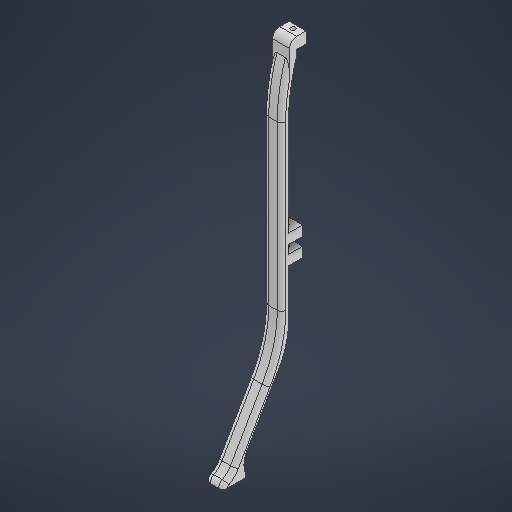
# Autodesk Inventor part: podpory
Saved by Autodesk Inventor 2026.2 (Build 302298010, 298A)
## iProperties
Created: 2026-04-19
Part Number: podpory
Material: Ogólny
Document SubType Name: Modeling
Designer: macie
Density: 1 g/cm^3
Appearance: Domyślna
Author: macie
Autodesk Inventor part; units mm, degrees
ref_plane "YZ Plane" through (0, 0, 0) normal (1, 0, 0) x (0, 1, 0)
ref_plane "XZ Plane" through (0, 0, 0) normal (0, 1, 0) x (-1, 0, 0)
ref_plane "XY Plane" through (0, 0, 0) normal (0, 0, 1) x (1, 0, 0)
sketch "Szkic1" plane through (0, 0, 0) normal (1, 0, 0) x (0, 1, 0)
  line L0 (0, 100.074) -> (0, 95.074)
  line L1 (0, 95.074) -> (5, 95.074)
  line L2 (5, 95.074) -> (5, 100.074)
  line L3 (5, 100.074) -> (0, 100.074)
  line L4 (178.8725, 94.2545) -> (173.8725, 94.2545)
  line L5 (173.8725, 94.2545) -> (173.8725, 89.2545)
  line L6 (173.8725, 89.2545) -> (178.8725, 89.2545)
  line L7 (178.8725, 89.2545) -> (178.8725, 94.2545)
  line L8 (5, 95.074) -> (137.3058, 95.074)
  arc A0 (173.8725, 89.2545) -> (137.3058, 95.074) centre (135.3654, -34.9115) ccw
  line L9 (5, 100.074) -> (137.3058, 100.074)
  arc A1 (173.8725, 94.2545) -> (137.3058, 100.074) centre (136.1596, -24.9207) ccw
  point P0 (0, 0)
  dimension "d0" = 95.074
  dimension "d1" = 5
  dimension "d2" = 5
  dimension "d4" = 0
  dimension "d5" = 89.2545
  dimension "d6" = 130
  dimension "d8" = 5
  dimension "d9" = 5
  dimension "d10" = 125
  dimension "d11" = 24.9207
  dimension "d12" = 34.9115
  dimension "d13" = 136.1596
  constraints: 20 end point, 4 parallel, 4 point on circle, 3 horizontal, 2 centre point, 2 perpendicular, 1 vertical
  measures "d0" distance from line of point (0, 0) L1
  measures "d1" distance between parallel lines of L1 L3
  measures "d2" distance between parallel lines of L0 L2
  measures "d4" distance from line of point (0, 0) L0
  measures "d5" distance from line of point (0, 0) L6
  measures "d6" radius of A0
  measures "d8" distance between parallel lines of L5 L7
  measures "d9" distance between parallel lines of L6 L4
  measures "d10" radius of A1
  measures "d11" vertical distance of point (0, 0) A1.centre
  measures "d12" vertical distance of point (0, 0) A0.centre
  measures "d13" horizontal distance of point (0, 0) A1.centre
extrude "Wyciągnięcie proste1" add sketch "Szkic1" along normal blind 12
sketch "Szkic2" plane through (0, 173.8725, 89.2545) normal (0, 0, -1) x (-1, 0, 0)
  line L0 (0, 0) -> (-12, 0) projected
  line L1 (0, 0) -> (-12, 0)
  line L2 (-12, 0) -> (-12, 12)
  line L3 (-12, 12) -> (0, 12)
  line L4 (0, 12) -> (0, 0)
  line L5 (-12, 0) -> (0, 0)
  line L6 (0, 0) -> (0, 4)
  line L7 (0, 4) -> (-12, 4)
  line L8 (-12, 4) -> (-12, 0)
  point P0 (0, -173.8725)
  point P1 (-12, 4)
  dimension "d16" = 12
  dimension "d17" = 12
  dimension "d18" = 4
  constraints: 16 end point, 4 parallel, 2 horizontal, 2 perpendicular, 1 point on line
  measures "d16" distance between parallel lines of L4 L2
  measures "d17" distance between parallel lines of L0 L3
  measures "d18" distance between parallel lines of L0 L7
extrude "Wyciągnięcie proste2" add sketch "Szkic2" along normal blind 6.653 and the other way blind 5 contours L7 L2 L3 L4
sketch "Szkic3" plane through (0, 177.8725, 89.2545) normal (0, -1, 0) x (1, 0, 0)
  line L0 (12, -6.653) -> (0, -6.653) projected
  line L1 (12, -6.653) -> (12, 5) projected
  line L2 (0, -6.653) -> (12, -6.653)
  line L3 (12, -6.653) -> (12, -3.5)
  line L4 (12, -3.5) -> (0, -3.5)
  line L5 (0, -3.5) -> (0, -6.653)
  line L6 (0, 0) -> (12, 0) projected
  point P0 (0, -89.2545)
  point P1 (6, -3.5)
  dimension "d50" = 3.5
  constraints: 8 end point, 2 parallel, 1 horizontal, 1 midpoint, 1 perpendicular, 1 point on line
  measures "d50" distance from line of L6 point (6, -3.5)
hole "Otwór1" at (6, 177.8725, 85.7545) direction (0, 1, 0) diameter 3.2 depth 8 tip angle 118
fillet "Zaokrąglenie1" radius 5 1 edges at (6, 185.8725, 94.2545)
sketch "Szkic5" plane through (0, 0, 95.074) normal (0, 0, -1) x (-1, 0, 0)
  line L0 (-12, 137.3058) -> (-12, 0) projected
  line L1 (-12, 67.8725) -> (0, 67.8725)
  line L2 (0, 67.8725) -> (0, 60.8725)
  line L3 (0, 60.8725) -> (-12, 60.8725)
  line L4 (-12, 60.8725) -> (-12, 67.8725)
  line L5 (-12, 177.8725) -> (0, 177.8725) projected
  line L6 (0, 137.3058) -> (0, 0) projected
  line L7 (-12, 54.7725) -> (0, 54.7725)
  line L8 (0, 54.7725) -> (0, 47.7725)
  line L9 (0, 47.7725) -> (-12, 47.7725)
  line L10 (-12, 47.7725) -> (-12, 54.7725)
  point P0 (0, 54.7725)
  dimension "d34" = 110
  dimension "d35" = 7
  dimension "d36" = 12
  dimension "d37" = 6.1
  dimension "d38" = 7
  constraints: 16 end point, 4 parallel, 3 point on line, 2 horizontal, 2 perpendicular
  measures "d34" distance between parallel lines of L1 L5
  measures "d35" distance between parallel lines of L3 L1
  measures "d36" distance between parallel lines of L0 L2
  measures "d37" distance between parallel lines of L7 L3
  measures "d38" distance between parallel lines of L7 L9
extrude "Wyciągnięcie proste3" add sketch "Szkic5" along normal blind 10 contours L1 L2 L3 L0 | L7 L6 L9 L0
sketch "Szkic6" plane through (0, 67.8725, 95.074) normal (0, 1, 0) x (1, 0, 0)
  line L0 (12, 0) -> (0, 0) projected
  line L1 (12, 0) -> (12, 10) projected
  point P0 (0, 95.074)
  point P1 (6, 4.326)
  point P2 (6, 0)
  dimension "d41" = 4.326
  dimension "d42" = 6
  constraints: 1 midpoint
  measures "d41" distance of point (6, 0) point (6, 4.326)
  measures "d42" distance from line of L1 point (6, 4.326)
hole "Otwór2" at (6, 67.8725, 90.748) direction (0, -1, 0) diameter 3.2 end through all
sketch "Szkic8" plane through (12, 0, 0) normal (1, 0, 0) x (0, 0, -1)
  line L0 (-100.074, 0) -> (-95.074, 0) projected
  line L1 (-95.074, 0) -> (-103.2542, -14.1684)
  line L2 (-100.074, 0) -> (-107.1294, -12.2203)
  line L3 (-100.074, 0) -> (-96.324, -2.1651)
  line L4 (-96.324, -2.1651) -> (-133.8518, -67.1651)
  line L5 (-133.8518, -67.1651) -> (-137.6018, -65)
  line L6 (-137.6018, -65) -> (-100.074, 0)
  line L7 (-141.6018, -67.1651) -> (-141.6018, -64.1651)
  line L8 (-141.6018, -64.1651) -> (-125.6018, -64.1651)
  line L9 (-125.6018, -64.1651) -> (-125.6018, -67.1651)
  line L10 (-125.6018, -67.1651) -> (-141.6018, -67.1651)
  point P0 (0, 0)
  point P1 (-133.6018, -67.1651)
  point P2 (-132.1197, -64.1651)
  point P3 (-137.1197, -64.1651)
  dimension "d53" = 60
  dimension "d54" = 60
  dimension "d55" = 65
  dimension "d56" = 3
  dimension "d57" = 4
  dimension "d58" = 8
  dimension "d59" = 0.8349
  constraints: 20 end point, 4 parallel, 3 perpendicular, 1 midpoint, 1 point on line, 1 vertical
  measures "d53" angle of L0 L1
  measures "d54" angle of L0 L2
  measures "d55" vertical distance of L4.end L3.end
  measures "d56" distance between parallel lines of L10 L8
  measures "d57" distance from line of L5.end L7
  measures "d58" distance from line of point (-133.602, -67.165) L9
  measures "d59" distance from line of L5.end L8
extrude "Wyciągnięcie proste5" add sketch "Szkic8" against normal blind 12
fillet "Zaokrąglenie2" radius 15 2 edges at (6, -64.1651, 132.1197) (6, -64.1651, 137.1197)
fillet "Zaokrąglenie3" radius 5 1 edges at (6, -64.1651, 141.6018)
fillet "Zaokrąglenie4" radius 80 1 edges at (6, 0, 100.074)
fillet "Zaokrąglenie5" radius 50 1 edges at (6, 0, 95.074)
fillet "Zaokrąglenie6" radius 3 12 edges at (0, 0.7304, 102.7999) (0, -37.975, 121.9989) (0, -60.6153, 135.7137) (0, -64.7693, 140.8322) (0, 79.3709, 100.074) (0, 155.8058, 98.5257) (12, 0.7304, 102.7999) (12, -37.975, 121.9989) (12, -60.6153, 135.7137) (12, -64.7693, 140.8322) (12, 79.3709, 100.074) (12, 155.8058, 98.5257)
equation "\"d38\" = d35"
equation "\"d54\" = d53"
